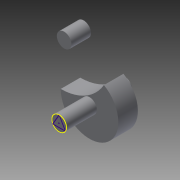
# Autodesk Inventor part: Geneva Drive
Saved by Autodesk Inventor 2018 (Build 220112000, 112)
## iProperties
Created: 2018-01-19
Part Number: Geneva Drive
Material: Generic
Document SubType Name: Modeling
Designer: Rus
Density: 1 g/cm^3
Appearance: Default
Mass: 42.38 g
Surface Area: 100.64 cm^2
Volume: 42.38 cm^3
Author: Rus
Autodesk Inventor part; units mm, degrees
ref_plane "YZ Plane" through (0, 0, 0) normal (1, 0, 0) x (0, 1, 0)
ref_plane "XZ Plane" through (0, 0, 0) normal (0, 1, 0) x (-1, 0, 0)
ref_plane "XY Plane" through (0, 0, 0) normal (0, 0, 1) x (1, 0, 0)
sketch "Sketch1" plane through (0, 0, 0) normal (0, 0, 1) x (1, 0, 0)
  line L0 (0, 0) -> (-87.9881, 0) construction
  line L1 (-87.9881, 0) -> (-21.9976, 38.1011) construction
  line L2 (-21.9976, 38.1011) -> (0, 0) construction
  arc A0 (-24.9453, 0) -> (12.4727, 21.6033) centre (0, 0) ccw
  line L3 (-24.9453, 0) -> (-24.9453, 43.2067) construction
  line L4 (-24.9453, 43.2067) -> (-21.9976, 38.1011) construction
  circle A1 centre (-21.9976, 38.1011) radius 6.35
  arc A2 (-24.9453, 0) -> (12.4727, 21.6033) centre (-24.9453, 43.2067) ccw
  dimension "d8" = 87.9881
  dimension "d9" = 43.9953
  dimension "d10" = 76.2
  dimension "d11" = 24.9453
  dimension "d12" = 12.7
  constraints: 10 end point, 4 coincident, 4 point on circle, 3 centre point, 1 collinear, 1 horizontal, 1 point on line, 1 vertical
  measures "d8" distance of L0.start L0.end
  measures "d9" distance of L1.end L0.start
  measures "d10" distance of L0.end L1.end
  measures "d11" radius of A0
  measures "d12" diameter of A1
extrude "Extrusion1" add sketch "Sketch1" along normal blind 16.9333
sketch "Sketch3" plane through (0, 0, 16.9333) normal (0, 0, 1) x (1, 0, 0)
  arc A0 (-24.9453, 0) -> (12.4727, 21.6033) centre (0, 0) ccw projected
  arc A1 (-24.9453, 0) -> (12.4727, 21.6033) centre (0, 0) ccw
  circle A2 centre (0, 0) radius 6.35
  arc A3 (-24.9453, 0) -> (12.4727, 21.6033) centre (-24.9453, 43.2067) ccw projected
  dimension "d30" = 12.7
  constraints: 2 centre point, 2 point on circle, 1 coincident, 1 concentric
  measures "d30" diameter of A2
extrude "Extrusion3" add sketch "Sketch3" along normal blind 26.416 and the other way blind 30.6493 contours A2
sketch "Sketch4" plane through (0, 0, 43.3493) normal (0, 0, 1) x (1, 0, 0)
  circle A0 centre (0, 0) radius 6.35 projected
  line L0 (0, 6.35) -> (5.4993, -3.175)
  line L1 (5.4993, -3.175) -> (-5.4993, -3.175)
  line L2 (-5.4993, -3.175) -> (0, 6.35)
  point P0 (0, 0)
  point P1 (0, 0)
  constraints: 6 end point, 1 coincident, 1 horizontal, 1 vertical alignment, 8 other
body "Solid1"
